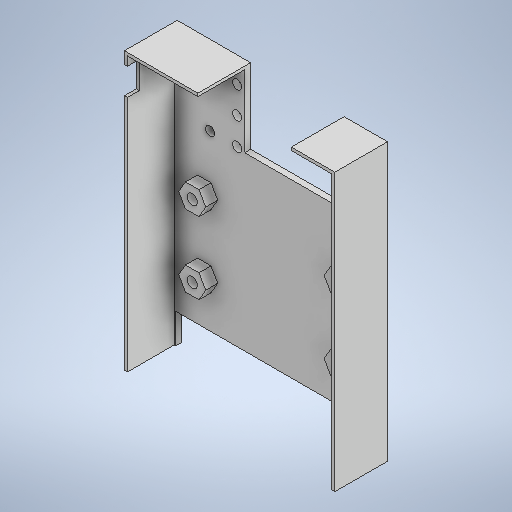
# Autodesk Inventor part: TES_Controller_V1_Case_Top
Saved by Autodesk Inventor 2025 (Build 290162000, 162)
## iProperties
Created: 2025-08-31
Part Number: TES_Controller_V1_Case_Top
Material: 常规
Document SubType Name: Modeling
Designer: 95052
Density: 1 g/cm^3
Appearance: 默认
Author: 95052
Autodesk Inventor part; units mm, degrees
ref_plane "YZ Plane" through (0, 0, 0) normal (1, 0, 0) x (0, 1, 0)
ref_plane "XZ Plane" through (0, 0, 0) normal (0, 1, 0) x (-1, 0, 0)
ref_plane "XY Plane" through (0, 0, 0) normal (0, 0, 1) x (1, 0, 0)
sketch "草图1" plane through (0, 0, 0) normal (0, 0, 1) x (1, 0, 0)
  line L0 (33.589, -45.4) -> (-33.589, -45.4)
  line L1 (-33.589, -45.4) -> (-33.589, 45.4)
  line L2 (-33.589, 45.4) -> (33.589, 45.4)
  line L3 (33.589, 45.4) -> (33.589, -45.4)
  line L4 (33.589, -45.4) -> (-33.589, 45.4) construction
  line L5 (-33.589, -45.4) -> (33.589, 45.4) construction
  line L6 (24.428, -20.313) -> (-24.072, -20.313) construction
  line L7 (-24.072, -20.313) -> (-24.072, 3.687) construction
  line L8 (-24.072, 3.687) -> (24.428, 3.687) construction
  line L9 (24.428, 3.687) -> (24.428, -20.313) construction
  line L10 (-22.3977, 6.587) -> (-20.7234, 3.687)
  line L11 (-20.7234, 3.687) -> (-22.3977, 0.787)
  line L12 (-22.3977, 0.787) -> (-25.7463, 0.787)
  line L13 (-25.7463, 0.787) -> (-27.4206, 3.687)
  line L14 (-27.4206, 3.687) -> (-25.7463, 6.587)
  line L15 (-25.7463, 6.587) -> (-22.3977, 6.587)
  line L16 (-22.3977, -17.413) -> (-20.7234, -20.313)
  line L17 (-20.7234, -20.313) -> (-22.3977, -23.213)
  line L18 (-22.3977, -23.213) -> (-25.7463, -23.213)
  line L19 (-25.7463, -23.213) -> (-27.4206, -20.313)
  line L20 (-27.4206, -20.313) -> (-25.7463, -17.413)
  line L21 (-25.7463, -17.413) -> (-22.3977, -17.413)
  line L22 (26.1023, -17.413) -> (27.7766, -20.313)
  line L23 (27.7766, -20.313) -> (26.1023, -23.213)
  line L24 (26.1023, -23.213) -> (22.7537, -23.213)
  line L25 (22.7537, -23.213) -> (21.0794, -20.313)
  line L26 (21.0794, -20.313) -> (22.7537, -17.413)
  line L27 (22.7537, -17.413) -> (26.1023, -17.413)
  line L28 (22.7537, 0.787) -> (21.0794, 3.687)
  line L29 (21.0794, 3.687) -> (22.7537, 6.587)
  line L30 (22.7537, 6.587) -> (26.1023, 6.587)
  line L31 (26.1023, 6.587) -> (27.7766, 3.687)
  line L32 (27.7766, 3.687) -> (26.1023, 0.787)
  line L33 (26.1023, 0.787) -> (22.7537, 0.787)
  point P0 (0, 0)
  point P1 (-24.072, -17.413)
  point P2 (24.428, -17.413)
  point P3 (24.428, 0.787)
  point P4 (24.428, 6.587)
  dimension "d0" = 90.8
  dimension "d1" = 67.178
  dimension "d2" = 25.087
  dimension "d3" = 9.161
  dimension "d4" = 9.517
  dimension "d5" = 41.713
  dimension "d6" = 2.9
  dimension "d7" = 2.9
  dimension "d8" = 2.9
  dimension "d9" = 2.9
  constraints: 68 end point, 6 midpoint, 4 coincident, 4 parallel, 3 point on line, 2 horizontal, 2 perpendicular, 52 other
  measures "d0" distance of L0.end L1.end
  measures "d1" distance of L0.start L0.end
  measures "d2" distance between parallel lines of L0 L6
  measures "d3" distance between parallel lines of L3 L9
  measures "d4" distance between parallel lines of L1 L7
  measures "d5" distance between parallel lines of L8 L2
  measures "d6" distance from line of L15 L7.end
  measures "d7" distance from line of L21 L6.end
  measures "d8" distance from line of L27 L6.start
  measures "d9" distance of point (24.428, 6.587) L8.end
extrude "拉伸1" add sketch "草图1" along normal blind 2
sketch "草图13" plane through (0, 0, 2) normal (0, 0, 1) x (1, 0, 0)
  line L0 (33.589, 45.4) -> (-33.589, 45.4) projected
  line L1 (-33.589, 45.4) -> (-33.589, -45.4) projected
  line L2 (-33.589, -45.4) -> (33.589, -45.4) projected
  line L3 (33.589, -45.4) -> (33.589, 45.4) projected
  line L4 (22.7537, 0.787) -> (21.0794, 3.687) projected
  line L5 (21.0794, 3.687) -> (22.7537, 6.587) projected
  line L6 (22.7537, 6.587) -> (26.1023, 6.587) projected
  line L7 (26.1023, 6.587) -> (27.7766, 3.687) projected
  line L8 (27.7766, 3.687) -> (26.1023, 0.787) projected
  line L9 (26.1023, 0.787) -> (22.7537, 0.787) projected
  line L10 (26.1023, -17.413) -> (27.7766, -20.313) projected
  line L11 (27.7766, -20.313) -> (26.1023, -23.213) projected
  line L12 (26.1023, -23.213) -> (22.7537, -23.213) projected
  line L13 (22.7537, -23.213) -> (21.0794, -20.313) projected
  line L14 (21.0794, -20.313) -> (22.7537, -17.413) projected
  line L15 (22.7537, -17.413) -> (26.1023, -17.413) projected
  line L16 (-22.3977, -17.413) -> (-20.7234, -20.313) projected
  line L17 (-20.7234, -20.313) -> (-22.3977, -23.213) projected
  line L18 (-22.3977, -23.213) -> (-25.7463, -23.213) projected
  line L19 (-25.7463, -23.213) -> (-27.4206, -20.313) projected
  line L20 (-27.4206, -20.313) -> (-25.7463, -17.413) projected
  line L21 (-25.7463, -17.413) -> (-22.3977, -17.413) projected
  line L22 (-22.3977, 6.587) -> (-20.7234, 3.687) projected
  line L23 (-20.7234, 3.687) -> (-22.3977, 0.787) projected
  line L24 (-22.3977, 0.787) -> (-25.7463, 0.787) projected
  line L25 (-25.7463, 0.787) -> (-27.4206, 3.687) projected
  line L26 (-27.4206, 3.687) -> (-25.7463, 6.587) projected
  line L27 (-25.7463, 6.587) -> (-22.3977, 6.587) projected
  line L28 (-19.5687, 3.687) -> (-21.8203, 7.587)
  line L29 (-21.8203, 7.587) -> (-26.3237, 7.587)
  line L30 (-26.3237, 7.587) -> (-28.5753, 3.687)
  line L31 (-28.5753, 3.687) -> (-26.3237, -0.213)
  line L32 (-26.3237, -0.213) -> (-21.8203, -0.213)
  line L33 (-21.8203, -0.213) -> (-19.5687, 3.687)
  line L34 (19.9247, 3.687) -> (22.1763, -0.213)
  line L35 (22.1763, -0.213) -> (26.6797, -0.213)
  line L36 (26.6797, -0.213) -> (28.9313, 3.687)
  line L37 (28.9313, 3.687) -> (26.6797, 7.587)
  line L38 (26.6797, 7.587) -> (22.1763, 7.587)
  line L39 (22.1763, 7.587) -> (19.9247, 3.687)
  line L40 (-19.5687, -20.313) -> (-21.8203, -16.413)
  line L41 (-21.8203, -16.413) -> (-26.3237, -16.413)
  line L42 (-26.3237, -16.413) -> (-28.5753, -20.313)
  line L43 (-28.5753, -20.313) -> (-26.3237, -24.213)
  line L44 (-26.3237, -24.213) -> (-21.8203, -24.213)
  line L45 (-21.8203, -24.213) -> (-19.5687, -20.313)
  line L46 (19.9247, -20.313) -> (22.1763, -24.213)
  line L47 (22.1763, -24.213) -> (26.6797, -24.213)
  line L48 (26.6797, -24.213) -> (28.9313, -20.313)
  line L49 (28.9313, -20.313) -> (26.6797, -16.413)
  line L50 (26.6797, -16.413) -> (22.1763, -16.413)
  line L51 (22.1763, -16.413) -> (19.9247, -20.313)
  point P0 (0, 0)
  dimension "d50" = 1
  dimension "d51" = 1
  dimension "d52" = 1
  dimension "d53" = 1
  constraints: 48 end point, 20 other
  measures "d50" distance between parallel lines of L22 L28
  measures "d51" distance between parallel lines of L4 L34
  measures "d52" distance between parallel lines of L16 L40
  measures "d53" distance between parallel lines of L13 L46
extrude "拉伸9" add sketch "草图13" along normal blind 0.5 contours L33 L32 L31 L30 L29 L28 | L39 L38 L37 L36 L35 L34 | L45 L44 L43 L42 L41 L40 | L51 L50 L49 L48 L47 L46
sketch "草图14" plane through (0, 0, 2.5) normal (0, 0, 1) x (1, 0, 0)
  line L0 (22.1763, -24.213) -> (19.9247, -20.313) projected
  line L1 (19.9247, -20.313) -> (22.1763, -16.413) projected
  line L2 (22.1763, -16.413) -> (26.6797, -16.413) projected
  line L3 (26.6797, -16.413) -> (28.9313, -20.313) projected
  line L4 (28.9313, -20.313) -> (26.6797, -24.213) projected
  line L5 (26.6797, -24.213) -> (22.1763, -24.213) projected
  line L6 (-21.8203, -16.413) -> (-19.5687, -20.313) projected
  line L7 (-19.5687, -20.313) -> (-21.8203, -24.213) projected
  line L8 (-21.8203, -24.213) -> (-26.3237, -24.213) projected
  line L9 (-26.3237, -24.213) -> (-28.5753, -20.313) projected
  line L10 (-28.5753, -20.313) -> (-26.3237, -16.413) projected
  line L11 (-26.3237, -16.413) -> (-21.8203, -16.413) projected
  line L12 (22.1763, -0.213) -> (19.9247, 3.687) projected
  line L13 (19.9247, 3.687) -> (22.1763, 7.587) projected
  line L14 (22.1763, 7.587) -> (26.6797, 7.587) projected
  line L15 (26.6797, 7.587) -> (28.9313, 3.687) projected
  line L16 (28.9313, 3.687) -> (26.6797, -0.213) projected
  line L17 (26.6797, -0.213) -> (22.1763, -0.213) projected
  line L18 (-21.8203, 7.587) -> (-19.5687, 3.687) projected
  line L19 (-19.5687, 3.687) -> (-21.8203, -0.213) projected
  line L20 (-21.8203, -0.213) -> (-26.3237, -0.213) projected
  line L21 (-26.3237, -0.213) -> (-28.5753, 3.687) projected
  line L22 (-28.5753, 3.687) -> (-26.3237, 7.587) projected
  line L23 (-26.3237, 7.587) -> (-21.8203, 7.587) projected
  line L24 (33.589, 45.4) -> (-33.589, 45.4) projected
  line L25 (-33.589, 45.4) -> (-33.589, -45.4) projected
  line L26 (-33.589, -45.4) -> (33.589, -45.4) projected
  line L27 (33.589, -45.4) -> (33.589, 45.4) projected
  circle A0 centre (-24.0693, 3.6854) radius 1.7
  circle A1 centre (24.428, 3.6854) radius 1.7
  circle A2 centre (24.428, -20.313) radius 1.7
  circle A3 centre (-24.0693, -20.313) radius 1.7
  point P0 (0, 0)
  dimension "d56" = 3.4
  dimension "d57" = 3.4
  dimension "d58" = 3.4
  dimension "d59" = 3.4
  constraints: 4 centre point
  measures "d56" diameter of A0
  measures "d57" diameter of A1
  measures "d58" diameter of A2
  measures "d59" diameter of A3
extrude "拉伸10" add sketch "草图14" along normal blind 3.5 contours L0 L1 L2 L3 L4 L5 | L6 L7 L8 L9 L10 L11 | L12 L13 L14 L15 L16 L17 | L18 L19 L20 L21 L22 L23
sketch "草图15" plane through (0, 0, 0) normal (0, 0, -1) x (-1, 0, 0)
  line L0 (-33.589, 45.4) -> (33.589, 45.4) projected
  line L1 (-20.589, 45.4) -> (10.589, 45.4)
  line L2 (10.589, 45.4) -> (10.589, 21.9)
  line L3 (10.589, 21.9) -> (-20.589, 21.9)
  line L4 (-20.589, 21.9) -> (-20.589, 45.4)
  line L5 (-33.589, -45.4) -> (-33.589, 45.4) projected
  line L6 (33.589, 45.4) -> (33.589, -45.4) projected
  point P0 (0, 0)
  dimension "d62" = 23.5
  dimension "d63" = 13
  dimension "d64" = 23
  constraints: 8 end point, 2 parallel, 1 horizontal, 1 perpendicular, 1 point on line
  measures "d62" distance between parallel lines of L0 L3
  measures "d63" distance between parallel lines of L5 L4
  measures "d64" distance between parallel lines of L6 L2
extrude "拉伸11" cut sketch "草图15" against normal blind 3.5
sketch "草图16" plane through (0, 0, 0) normal (0, 0, -1) x (-1, 0, 0)
  circle A0 centre (-26.0747, 39.6778) radius 2.5
  circle A1 centre (-26.0747, 33.1778) radius 2.5
  circle A2 centre (-26.0747, 26.6778) radius 2.5
  line L0 (-26.0747, 39.6778) -> (-26.0747, 26.6778) construction
  point P0 (0, 0)
  dimension "d67" = 5
  dimension "d68" = 5
  dimension "d69" = 5
  dimension "d70" = 6.5
  dimension "d71" = 6.5
  constraints: 3 centre point, 2 end point, 2 vertical alignment, 1 vertical
  measures "d67" diameter of A0
  measures "d68" diameter of A1
  measures "d69" diameter of A2
  measures "d70" distance of A1.centre L0.start
  measures "d71" distance of L0.end A1.centre
extrude "拉伸12" cut sketch "草图16" against normal through all
sketch "草图17" plane through (0, 0, 0) normal (0, 0, -1) x (-1, 0, 0)
  line L0 (33.589, -45.4) -> (-33.589, -45.4) projected
  line L1 (33.589, 45.4) -> (33.589, -45.4) projected
  line L2 (-33.589, -45.4) -> (33.589, -45.4)
  line L3 (33.589, -45.4) -> (33.589, -35.4)
  line L4 (33.589, -35.4) -> (-33.589, -35.4)
  line L5 (-33.589, -35.4) -> (-33.589, -45.4)
  point P0 (0, 0)
  dimension "d74" = 10
  constraints: 8 end point, 2 parallel, 1 horizontal, 1 perpendicular, 1 point on line
  measures "d74" distance between parallel lines of L0 L4
sketch "草图18" plane through (0, 0, 0) normal (0, 0, -1) x (-1, 0, 0)
  circle A0 centre (-26.0747, 26.6778) radius 2.5 projected
  circle A1 centre (-26.0747, 33.1778) radius 2.5 projected
  circle A2 centre (-26.0747, 39.6778) radius 2.5 projected
  line L0 (22.3977, 6.587) -> (20.7234, 3.687) projected
  line L1 (25.7463, 6.587) -> (22.3977, 6.587) projected
  line L2 (27.4206, 3.687) -> (25.7463, 6.587) projected
  line L3 (25.7463, 0.787) -> (27.4206, 3.687) projected
  line L4 (22.3977, 0.787) -> (25.7463, 0.787) projected
  line L5 (20.7234, 3.687) -> (22.3977, 0.787) projected
  line L6 (22.3977, -17.413) -> (20.7234, -20.313) projected
  line L7 (25.7463, -17.413) -> (22.3977, -17.413) projected
  line L8 (27.4206, -20.313) -> (25.7463, -17.413) projected
  line L9 (25.7463, -23.213) -> (27.4206, -20.313) projected
  line L10 (22.3977, -23.213) -> (25.7463, -23.213) projected
  line L11 (20.7234, -20.313) -> (22.3977, -23.213) projected
  line L12 (-26.1023, -17.413) -> (-27.7766, -20.313) projected
  line L13 (-22.7537, -17.413) -> (-26.1023, -17.413) projected
  line L14 (-21.0794, -20.313) -> (-22.7537, -17.413) projected
  line L15 (-22.7537, -23.213) -> (-21.0794, -20.313) projected
  line L16 (-26.1023, -23.213) -> (-22.7537, -23.213) projected
  line L17 (-27.7766, -20.313) -> (-26.1023, -23.213) projected
  line L18 (-22.7537, 0.787) -> (-21.0794, 3.687) projected
  line L19 (-26.1023, 0.787) -> (-22.7537, 0.787) projected
  line L20 (-27.7766, 3.687) -> (-26.1023, 0.787) projected
  line L21 (-26.1023, 6.587) -> (-27.7766, 3.687) projected
  line L22 (-22.7537, 6.587) -> (-26.1023, 6.587) projected
  line L23 (-21.0794, 3.687) -> (-22.7537, 6.587) projected
  line L24 (10.589, 45.4) -> (10.589, 21.9) projected
  line L25 (10.589, 21.9) -> (-20.589, 21.9) projected
  line L26 (-20.589, 21.9) -> (-20.589, 45.4) projected
  line L27 (-33.589, 45.4) -> (-20.589, 45.4) projected
  line L28 (-33.589, -45.4) -> (-33.589, 45.4) projected
  line L29 (33.589, -45.4) -> (-33.589, -45.4) projected
  line L30 (33.589, 45.4) -> (33.589, -45.4) projected
  line L31 (10.589, 45.4) -> (33.589, 45.4) projected
  line L32 (10.589, 45.9) -> (34.089, 45.9)
  line L33 (34.089, 45.9) -> (34.089, -45.4)
  line L34 (-34.089, -45.4) -> (-34.089, 45.9)
  line L35 (-34.089, 45.9) -> (-20.589, 45.9)
  line L36 (-33.589, -45.4) -> (-34.089, -45.4)
  line L37 (33.589, -45.4) -> (34.089, -45.4)
  line L38 (-20.589, 45.4) -> (-20.589, 45.9)
  line L39 (10.589, 45.4) -> (10.589, 45.9)
  point P0 (0, 0)
  constraints: 16 end point, 2 perpendicular, 1 parallel, 1 point on line
extrude "拉伸13" add sketch "草图18" against normal up to surface (2 mm away) contours L39 L32 L33 L37 L30 L31 | L27 L28 L36 L34 L35 L38
extrude "拉伸14" cut sketch "草图17" against normal through all
sketch "草图19" plane through (0, 0, 0) normal (0, 0, -1) x (-1, 0, 0)
  line L0 (-33.589, -45.4) -> (-33.589, -35.4) projected
  line L1 (-33.589, -35.4) -> (33.589, -35.4) projected
  line L2 (33.589, -35.4) -> (33.589, -45.4) projected
  line L3 (33.589, -45.4) -> (34.089, -45.4) projected
  line L4 (34.089, -45.4) -> (34.089, 45.9) projected
  line L5 (34.089, 45.9) -> (10.589, 45.9) projected
  line L6 (10.589, 45.9) -> (10.589, 21.9) projected
  line L7 (10.589, 21.9) -> (-20.589, 21.9) projected
  line L8 (-20.589, 21.9) -> (-20.589, 45.9) projected
  line L9 (-20.589, 45.9) -> (-34.089, 45.9) projected
  line L10 (-34.089, 45.9) -> (-34.089, -45.4) projected
  line L11 (-34.089, -45.4) -> (-33.589, -45.4) projected
  line L12 (-22.7537, 0.787) -> (-21.0794, 3.687) projected
  line L13 (-26.1023, 0.787) -> (-22.7537, 0.787) projected
  line L14 (-27.7766, 3.687) -> (-26.1023, 0.787) projected
  line L15 (-26.1023, 6.587) -> (-27.7766, 3.687) projected
  line L16 (-22.7537, 6.587) -> (-26.1023, 6.587) projected
  line L17 (-21.0794, 3.687) -> (-22.7537, 6.587) projected
  line L18 (-26.1023, -17.413) -> (-27.7766, -20.313) projected
  line L19 (-22.7537, -17.413) -> (-26.1023, -17.413) projected
  line L20 (-21.0794, -20.313) -> (-22.7537, -17.413) projected
  line L21 (-22.7537, -23.213) -> (-21.0794, -20.313) projected
  line L22 (-26.1023, -23.213) -> (-22.7537, -23.213) projected
  line L23 (-27.7766, -20.313) -> (-26.1023, -23.213) projected
  line L24 (22.3977, -17.413) -> (20.7234, -20.313) projected
  line L25 (25.7463, -17.413) -> (22.3977, -17.413) projected
  line L26 (27.4206, -20.313) -> (25.7463, -17.413) projected
  line L27 (25.7463, -23.213) -> (27.4206, -20.313) projected
  line L28 (22.3977, -23.213) -> (25.7463, -23.213) projected
  line L29 (20.7234, -20.313) -> (22.3977, -23.213) projected
  line L30 (22.3977, 6.587) -> (20.7234, 3.687) projected
  line L31 (25.7463, 6.587) -> (22.3977, 6.587) projected
  line L32 (27.4206, 3.687) -> (25.7463, 6.587) projected
  line L33 (25.7463, 0.787) -> (27.4206, 3.687) projected
  line L34 (22.3977, 0.787) -> (25.7463, 0.787) projected
  line L35 (20.7234, 3.687) -> (22.3977, 0.787) projected
  circle A0 centre (-26.0747, 39.6778) radius 2.5 projected
  circle A1 centre (-26.0747, 33.1778) radius 2.5 projected
  circle A2 centre (-26.0747, 26.6778) radius 2.5 projected
  line L36 (-35.089, -45.4) -> (-35.089, 46.9)
  line L37 (-35.089, 46.9) -> (-20.589, 46.9)
  line L38 (10.589, 46.9) -> (35.089, 46.9)
  line L39 (35.089, 46.9) -> (35.089, -45.4)
  line L40 (-34.089, -45.4) -> (-35.089, -45.4)
  line L41 (34.089, -45.4) -> (35.089, -45.4)
  line L42 (-20.589, 45.9) -> (-20.589, 46.9)
  line L43 (10.589, 45.9) -> (10.589, 46.9)
  point P0 (0, 0)
  constraints: 16 end point, 2 perpendicular, 1 parallel, 1 point on line
extrude "拉伸15" add sketch "草图19" against normal blind 17.6 contours L40 L36 L37 L42 L9 L10 | L4 L5 L43 L38 L39 L41
sketch "草图20" plane through (0, 0, 0) normal (0, 0, -1) x (-1, 0, 0)
  line L0 (12.089, 45.793) -> (12.089, 23.9831) construction
  line L1 (10.589, 46.9) -> (10.589, 21.9) construction
  line L2 (13.089, 45.793) -> (13.089, 23.9831) construction
  circle A0 centre (13.089, 40.4) radius 1.5
  circle A1 centre (13.089, 31.4) radius 1.5
  circle A2 centre (13.089, 22.4) radius 1.5
  line L3 (35.089, 46.9) -> (10.589, 46.9) projected
  circle A3 centre (22.089, 22.4) radius 1.5
  point P0 (0, 0)
  dimension "d83" = 1.5
  dimension "d84" = 1
  dimension "d85" = 3
  dimension "d86" = 3
  dimension "d87" = 3
  dimension "d88" = 9
  dimension "d89" = 9
  dimension "d90" = 6.5
  dimension "d91" = 3
  dimension "d92" = 9
  constraints: 4 centre point, 4 end point, 3 point on line, 1 parallel, 1 vertical
  measures "d83" distance between parallel lines of L1 L0
  measures "d84" distance between parallel lines of L0 L2
  measures "d85" diameter of A0
  measures "d86" diameter of A1
  measures "d87" diameter of A2
  measures "d88" distance of A1.centre A0.centre
  measures "d89" distance of A2.centre A1.centre
  measures "d90" distance from line of L3 A0.centre
  measures "d91" diameter of A3
  measures "d92" distance of A2.centre A3.centre
extrude "拉伸16" cut sketch "草图20" against normal through all
sketch "草图21" plane through (-35.089, -45.4, 0) normal (-1, 0, 0) x (0, 0, 1)
  line L0 (17.6, 92.3) -> (17.6, 0) construction
  line L1 (17.6, 90.8) -> (0, 90.8) construction
  line L2 (0, 92.3) -> (17.6, 92.3) construction
  line L3 (17.6, 88.3) -> (13.6, 88.3)
  line L4 (13.6, 88.3) -> (13.6, 79.3)
  line L5 (13.6, 79.3) -> (17.6, 79.3)
  line L6 (17.6, 79.3) -> (17.6, 88.3)
  point P0 (0, 45.4)
  point P1 (15.6, 79.3)
  dimension "d95" = 1.5
  dimension "d96" = 2.5
  dimension "d97" = 4
  dimension "d98" = 9
  constraints: 10 end point, 2 parallel, 2 perpendicular, 2 point on line, 1 horizontal, 1 midpoint
  measures "d95" distance between parallel lines of L2 L1
  measures "d96" distance between parallel lines of L1 L3
  measures "d97" distance between parallel lines of L0 L4
  measures "d98" distance from line of point (15.6, 79.3) L3
extrude "拉伸17" cut sketch "草图21" against normal up to surface (1 mm away)
